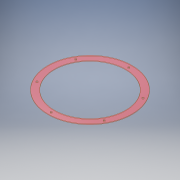
# Autodesk Inventor part: Bearing Spacer
Saved by Autodesk Inventor 2019.4 (Build 234330000, 330)
## iProperties
Created: 2020-01-23
Part Number: Bearing Spacer
Material: Polycarbonate, Smoke
Document SubType Name: Modeling
Designer: admin
Density: 1.2 g/cm^3
Appearance: Polycarbonate - Smoked
Author: admin
Autodesk Inventor part; units mm, degrees
ref_plane "YZ Plane" through (0, 0, 0) normal (1, 0, 0) x (0, 1, 0)
ref_plane "XZ Plane" through (0, 0, 0) normal (0, 1, 0) x (-1, 0, 0)
ref_plane "XY Plane" through (0, 0, 0) normal (0, 0, 1) x (1, 0, 0)
sketch "Sketch1" plane through (0, 0, 0) normal (0, 1, 0) x (-1, 0, 0)
  circle A0 centre (0, 0) radius 175
  circle A1 centre (0, 0) radius 148
  line L0 (0, 161.5) -> (139.8631, 80.75) construction
  line L1 (139.8631, 80.75) -> (139.8631, -80.75) construction
  line L2 (139.8631, -80.75) -> (0, -161.5) construction
  line L3 (0, -161.5) -> (-139.8631, -80.75) construction
  line L4 (-139.8631, -80.75) -> (-139.8631, 80.75) construction
  line L5 (-139.8631, 80.75) -> (0, 161.5) construction
  circle A2 centre (139.8631, -80.75) radius 3.5
  circle A3 centre (139.8631, 80.75) radius 3.5
  circle A4 centre (0, 161.5) radius 3.5
  circle A5 centre (-139.8631, 80.75) radius 3.5
  circle A6 centre (-139.8631, -80.75) radius 3.5
  circle A7 centre (0, -161.5) radius 3.5
  dimension "d0" = 350
  dimension "d1" = 27
  dimension "d2" = 7
  dimension "d3" = 7
  dimension "d4" = 7
  dimension "d5" = 7
  dimension "d6" = 7
  dimension "d7" = 7
  dimension "d8" = 323
  constraints: 12 end point, 9 coincident, 8 centre point, 1 vertical, 13 other
  measures "d0" diameter of A0
  measures "d1" radial gap between concentric circles of A0 A1
  measures "d2" diameter of A2
  measures "d3" diameter of A3
  measures "d4" diameter of A4
  measures "d5" diameter of A5
  measures "d6" diameter of A6
  measures "d7" diameter of A7
  measures "d8" distance of A4.centre A7.centre
extrude "Extrusion1" add sketch "Sketch1" along normal blind 3
equation "\"d8\" = d0 - d1"
body "Solid1"
